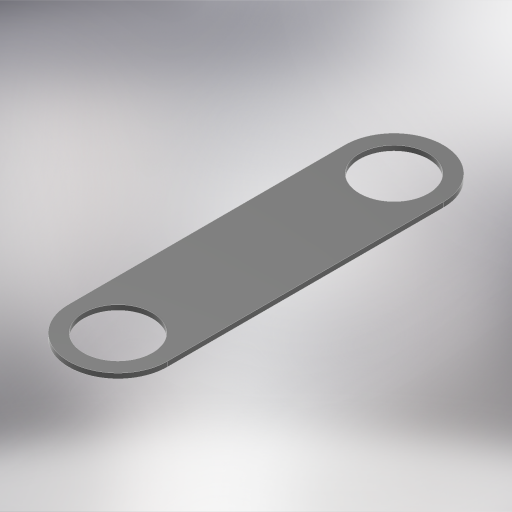
# Autodesk Inventor part: intake 1.1
Saved by Autodesk Inventor 2023 (Build 270158000, 158)
## iProperties
Created: 2023-07-16
Part Number: intake 1.1
Material: Acetal Resin, Black
Document SubType Name: Modeling
Designer: aaron
Density: 1.425 g/cm^3
Appearance: Smooth - Black
Author: aaron
Autodesk Inventor part; units mm, degrees
ref_plane "YZ Plane" through (0, 0, 0) normal (1, 0, 0) x (0, 1, 0)
ref_plane "XZ Plane" through (0, 0, 0) normal (0, 1, 0) x (-1, 0, 0)
ref_plane "XY Plane" through (0, 0, 0) normal (0, 0, 1) x (1, 0, 0)
sketch "Sketch1" plane through (0, 0, 0) normal (0, 1, 0) x (-1, 0, 0)
  circle A0 centre (0, 0) radius 11.1125
  circle A1 centre (0, 0) radius 15.875
  line L0 (0, 0) -> (0, 88.9) construction
  line L1 (-15.875, 0) -> (-15.875, 88.9)
  line L2 (15.875, 88.9) -> (15.875, 0)
  arc A2 (-15.875, 0) -> (15.875, 0) centre (0, 0) ccw
  arc A3 (15.875, 88.9) -> (-15.875, 88.9) centre (0, 88.9) ccw
  circle A4 centre (0, 88.9) radius 11.1125
  point P0 (0, 44.45)
  dimension "d0" = 22.225
  dimension "d1" = 31.75
  dimension "d2" = 88.9
  dimension "d3" = 22.225
  constraints: 8 end point, 5 centre point, 4 point on circle, 4 tangent, 3 coincident, 1 concentric, 1 midpoint, 1 parallel, 1 vertical
  measures "d0" diameter of A0
  measures "d1" diameter of A1
  measures "d2" distance of L0.end point (0, 0)
  measures "d3" diameter of A4
extrude "Extrusion1" add sketch "Sketch1" along normal blind 1.5875
body "Solid1"
